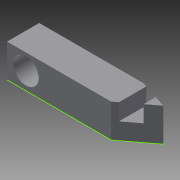
# Autodesk Inventor part: hook
Saved by Autodesk Inventor 2015 (Build 190159000, 159)
## iProperties
Created: 2015-01-12
Part Number: hook
Material: Nylon 6/6
Document SubType Name: Modeling
Designer: whitaus15
Density: 1.13 g/cm^3
Appearance: Nylon 6
Author: whitaus15
Autodesk Inventor part; units mm, degrees
ref_plane "YZ Plane" through (0, 0, 0) normal (1, 0, 0) x (0, 1, 0)
ref_plane "XZ Plane" through (0, 0, 0) normal (0, 1, 0) x (-1, 0, 0)
ref_plane "XY Plane" through (0, 0, 0) normal (0, 0, 1) x (1, 0, 0)
sketch "Sketch1" plane through (0, 0, 0) normal (0, 1, 0) x (-1, 0, 0)
  line L0 (0, 2.4651) -> (7.9791, 2.4651)
  line L1 (7.9791, 2.4651) -> (7.9791, 0)
  line L2 (7.9791, 0) -> (0, 0)
  line L3 (0, 0) -> (0, 2.4651)
  line L4 (0, 0) -> (-2.2705, 0.7352)
  line L5 (-2.2705, 0.7352) -> (0, 2.4651)
  constraints: 12 end point, 3 perpendicular, 1 horizontal
extrude "Extrusion1" add sketch "Sketch1" along normal blind 2.54 contours L0 L1 L2 L3
extrude "Extrusion2" add sketch "Sketch1" along normal blind 2.54 contours L3 L4 L5
sketch "Sketch2" plane through (0, 2.54, 0) normal (0, 1, 0) x (1, 0, 0)
  line L0 (0, -2.4651) -> (2.2705, -0.7352) projected
  line L1 (0.3368, -2.2085) -> (0.3368, -0.1091)
  line L2 (2.2705, -0.7352) -> (0, 0) projected
  line L3 (1.4116, -0.4571) -> (1.4116, -1.3896)
  line L4 (0.3368, -2.2085) -> (1.4116, -1.3896)
  line L5 (0.3368, -0.1091) -> (1.4116, -0.4571)
  line L6 (0.3368, -2.2085) -> (1.4116, -1.3896)
  constraints: 10 end point, 4 point on line, 3 collinear, 1 parallel, 1 vertical
extrude "Extrusion3" cut sketch "Sketch2" against normal blind 1.27 contours L1 L2 L3 L0
sketch "Sketch3" plane through (-7.9791, 0, 2.4651) normal (0, 0, 1) x (1, 0, 0)
  circle A0 centre (1.4488, 1.319) radius 0.9757
  point P0 (7.9791, 0)
  constraints: 1 centre point
extrude "Extrusion4" cut sketch "Sketch3" against normal blind 5.08
body "Solid1"
